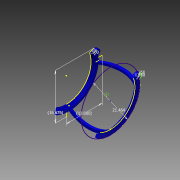
# Autodesk Inventor part: Outer
Saved by Autodesk Inventor 2014 (Build 180170000, 170)
## iProperties
Created: 2014-01-05
Part Number: Outer
Material: Polystyrene
Document SubType Name: Modeling
Designer: Tristan Debrunner
Density: 1.1072 g/cm^3
Appearance: Smooth - White
Mass: 1385.31 g
Surface Area: 1960.58 cm^2
Volume: 1251.19 cm^3
Author: Tristan Debrunner
Autodesk Inventor part; units mm, degrees
ref_plane "YZ Plane" through (0, 0, 0) normal (1, 0, 0) x (0, 1, 0)
ref_plane "XY Plane" through (0, 0, 0) normal (0, 0, 1) x (1, 0, 0)
sketch "Sketch1" plane through (0, 0, 0) normal (0, 0, 1) x (1, 0, 0)
  line L0 (0, 0) -> (0, -45.7841)
  line L1 (25.4, -20.3841) -> (25.4, -45.7841)
  arc A0 (0, 0) -> (25.4, -20.3841) centre (203.2, 227.1845) ccw
  line L2 (25.4, -45.7841) -> (0, -45.7841)
  line L3 (406.4, 0) -> (406.4, -45.7841)
  line L4 (381, -20.3841) -> (381, -45.7841)
  arc A1 (381, -20.3841) -> (406.4, 0) centre (203.2, 227.1845) ccw
  line L5 (381, -45.7841) -> (406.4, -45.7841)
  line L6 (0, 227.1845) -> (560.8643, 227.1845)
  constraints: 14 end point, 4 point on circle, 2 centre point, 2 vertical, 1 perpendicular
revolve "Revolution1" add sketch "Sketch1" angle 110 about axis through (0, 227.1845, 0) along (1, 0, 0)
sketch "Sketch2" plane through (381, -45.7841, 0) normal (0, 0, 1) x (1, 0, 0)
  line L0 (0, 0) -> (0, 25.4) projected
  line L1 (-381, 45.7841) -> (-381, 0) projected
  line L2 (-381, 0) -> (-355.6, 0) projected
  line L3 (-355.6, 0) -> (-355.6, 25.4) projected
  arc A0 (-381, 45.7841) -> (-355.6, 25.4) centre (-177.8, 272.9686) ccw projected
  arc A1 (-355.6, 25.4) -> (0, 25.4) centre (-177.8, 272.9686) ccw
  arc A2 (-355.6, 0) -> (0, 0) centre (-177.8, 247.5686) ccw
  line L4 (0, 0) -> (0, 25.4)
  line L5 (-355.6, 25.4) -> (-355.6, 0)
  line L6 (-177.8, 272.9686) -> (227.4781, 272.9686)
  dimension "d6" = 304.8
  constraints: 6 end point, 4 point on circle, 2 centre point, 2 collinear, 2 point on line, 1 parallel
  measures "d6" radius of A2
revolve "Revolution2" add sketch "Sketch2" angle 4 about axis through (203.2, 227.1845, 0) along (1, 0, 0) contours A2 L3 A1 L0
ref_plane "Work Plane1" through (0, 304.8, 0) normal (0, 1, 0) x (-1, 0, 0)
ref_plane "Work Plane2" through (560.8643, 227.1845, 0) normal (0, 1, 0) x (-1, 0, 0)
sketch "Sketch5" plane through (560.8643, 227.1845, 0) normal (0, 1, 0) x (-1, 0, 0)
  arc A0 (154.4643, -227.1845) -> (179.8643, -247.5686) centre (357.6643, 0) ccw projected
  line L0 (179.8643, -247.5686) -> (179.8643, -272.9686) projected
  line L1 (179.8643, -272.9686) -> (154.4643, -272.9686) projected
  line L2 (154.4643, -272.9686) -> (154.4643, -227.1845) projected
  line L3 (535.4643, -272.9686) -> (535.4643, -247.5686) projected
  line L4 (560.8643, -227.1845) -> (560.8643, -272.9686) projected
  line L5 (560.8643, -272.9686) -> (535.4643, -272.9686) projected
  arc A1 (179.8643, -247.5686) -> (535.4643, -247.5686) centre (357.6643, 0) ccw
  arc A2 (179.8643, -272.9686) -> (535.4643, -272.9686) centre (357.6643, -25.4) ccw
  line L6 (179.8643, -272.9686) -> (179.8643, -247.5686)
  line L7 (535.4643, -272.9686) -> (535.4643, -247.5686)
  line L8 (357.6643, 0) -> (560.8643, 0)
  arc A3 (535.4643, -247.5686) -> (560.8643, -227.1845) centre (357.6643, 0) ccw projected
  dimension "d30" = 304.8
  dimension "d31" = 304.8
  constraints: 6 end point, 4 point on circle, 2 centre point, 2 equal length
  measures "d30" radius of A1
  measures "d31" radius of A2
revolve "Revolution4" add sketch "Sketch5" angle 4 about axis through (203.2, 227.1845, 0) along (-1, 0, 0) contours A1 L3 A2 L0
sketch "Sketch6" plane through (25.4, 227.1845, -247.5686) normal (1, 0, 0) x (0, 0, -1)
  line L0 (0, 0) -> (25.4, 0) projected
  line L1 (-14.9302, 84.6734) -> (8.938, 93.3608) projected
  line L2 (-2.9961, 89.0171) -> (-2.9961, 76.3171)
  point P0 (-247.5686, -227.1845)
  dimension "d33" = 12.7
  constraints: 2 end point, 1 midpoint, 1 perpendicular
  measures "d33" distance of L2.start L2.end
sketch3d "3D Sketch2"
sketch "Sketch7" plane through (0, -45.7841, 0) normal (-1, 0, 0) x (0, 0, 1)
  circle A0 centre (-244.5725, 349.2857) radius 3.175 projected
  line L0 (0, 45.7841) -> (0, 0) projected
  arc A1 (-213.4836, 350.6703) -> (0, 45.7841) centre (0, 272.9686) ccw projected
  line L1 (-256.5066, 366.3293) -> (-213.4836, 350.6703) projected
  arc A2 (-256.5066, 366.3293) -> (0, 0) centre (0, 272.9686) ccw projected
  line L2 (-272.9686, 272.9686) -> (-330.2, 272.9686) projected
  line L3 (0, -57.2314) -> (0, 0) projected
  dimension "d48" = 423.5607
  dimension "d49" = 330.2
  measures "d48" vertical distance of L3.start L1.start
  measures "d49" horizontal distance of L2.end L3.start
revolve "Revolution5" add sketch "Sketch1" angle 25 about axis through (0, 227.1845, 0) along (-1, 0, 0)
sketch "Sketch8" plane through (406.4, 304.8862, -213.4836) normal (1, 0, 0) x (0, 0.3420201, -0.9396926)
  arc A0 (-420.2024, -193.0179) -> (45.7841, 0) centre (-227.1845, 0) ccw projected
  arc A1 (-387.8282, -160.6437) -> (0, 0) centre (-227.1845, 0) ccw projected
  circle A2 centre (-227.1845, 0) radius 272.5928
  arc A3 (41.0575, -50.5776) -> (45.7841, 0) centre (43.1926, -25.2675) ccw
  arc A4 (41.0575, -50.5776) -> (45.7841, 0) centre (-227.1845, 0) ccw
  circle A5 centre (44.2224, -25.399) radius 3.175
  point P0 (-304.8862, -213.4836)
  dimension "d51" = 545.1856
  dimension "d52" = 25.4
  dimension "d53" = 6.35
  constraints: 5 point on circle, 3 centre point, 1 coincident, 1 concentric, 3 other
  measures "d52" radius of A3
  measures "d53" diameter of A5
extrude "Extrusion1" add sketch "Sketch8" against normal blind 25.4 contours A0 A5 A3 | A0 A5
sketch "Sketch9" plane through (0, 320.5453, -256.5066) normal (-1, 0, 0) x (0, -0.3420201, 0.9396926)
  arc A0 (0, 0) -> (465.9865, -193.0179) centre (272.9686, 0) ccw projected
  arc A1 (0, 0) -> (4.7266, -50.5776) centre (2.5915, -25.2675) ccw projected
  point P0 (350.6703, -213.4836)
extrude "Extrusion2" add sketch "Sketch9" against normal blind 25.4
extrude "Extrusion3" cut sketch "Sketch8" against normal through all contours A5 A2 A0 | A0 A5 | A5 A2 picked at (43.1631, -25.4275)
body "Solid1"
